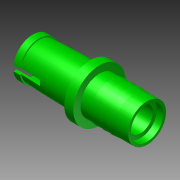
# Autodesk Inventor part: T9 Axle
Saved by Autodesk Inventor 2015 (Build 190159000, 159)
## iProperties
Created: 2012-02-20
Part Number: T9 Axle
Material: Generic
Document SubType Name: Modeling
Designer: Thom Tremblay
Density: 1 g/cm^3
Appearance: Dark Green
Author: Thom Tremblay
Autodesk Inventor part; units mm, degrees
ref_plane "YZ Plane" through (0, 0, 0) normal (1, 0, 0) x (0, 1, 0)
ref_plane "XZ Plane" through (0, 0, 0) normal (0, 1, 0) x (-1, 0, 0)
ref_plane "XY Plane" through (0, 0, 0) normal (0, 0, 1) x (1, 0, 0)
sketch "Sketch1" plane through (0, 0, 0) normal (0, 0, 1) x (1, 0, 0)
  line L0 (0, 0) -> (1.778, 0)
  line L1 (1.778, 0) -> (1.778, 5.08)
  line L2 (1.778, 5.08) -> (0, 5.08)
  line L3 (0, 5.08) -> (0, 0)
  line L4 (1.778, 0) -> (11.049, 0)
  line L5 (11.049, 0) -> (11.049, 3.683)
  line L6 (11.049, 3.683) -> (1.778, 3.683)
  line L7 (1.778, 3.683) -> (1.778, 0)
  line L8 (8.509, 3.683) -> (6.985, 3.81)
  line L9 (6.985, 3.81) -> (6.985, 3.683)
  line L10 (6.985, 3.683) -> (5.461, 3.81)
  line L11 (5.461, 3.81) -> (5.461, 3.683)
  line L12 (5.461, 3.683) -> (3.937, 3.81)
  line L13 (3.937, 3.81) -> (3.937, 3.683)
  line L14 (0, 0) -> (0, 3.1252)
  line L15 (0, 3.81) -> (0.889, 3.81) construction
  line L16 (0, 3.81) -> (0, 0)
  arc A0 (0, 3.81) -> (-9.906, 3.556) centre (0, -189.484) ccw
  line L17 (-9.906, 3.556) -> (-9.906, 3.81)
  line L18 (-9.906, 3.81) -> (-11.176, 3.81)
  line L19 (-11.176, 3.81) -> (-11.176, 0)
  line L20 (-11.176, 0) -> (0, 0)
  dimension "d0" = 1.778
  dimension "d1" = 10.16
  dimension "d2" = 9.271
  dimension "d3" = 7.366
  dimension "d4" = 7.62
  dimension "d5" = 2.54
  dimension "d6" = 1.524
  dimension "d7" = 7.62
  dimension "d8" = 7.62
  dimension "d9" = 11.176
  dimension "d10" = 7.112
  dimension "d11" = 1.27
  constraints: 42 end point, 8 parallel, 7 perpendicular, 6 point on line, 2 collinear, 2 horizontal, 2 horizontal alignment, 2 point on circle, 1 centre point, 1 tangent
  measures "d0" distance of L1.end L2.end
  measures "d1" diameter of L2 L0
  measures "d2" distance of L5.end L6.end
  measures "d3" diameter of L6 L4
  measures "d4" diameter of L8.end L4
  measures "d5" distance of L5.end L8.start
  measures "d6" horizontal distance of L8.start L8.end
  measures "d7" diameter of L18 L20
  measures "d8" diameter of L15 L20
  measures "d9" distance of L19.end L0.start
  measures "d10" diameter of L17.start L20
  measures "d11" distance of L17.end L18.end
revolve "Revolution1" add sketch "Sketch1" angle 360 about axis through (-11.176, 0, 0) along (1, 0, 0)
sketch "Sketch2" plane through (0, 0, 0) normal (0, 0, 1) x (1, 0, 0)
  line L0 (-11.176, 0.508) -> (-6.096, 0.508)
  line L1 (-6.096, 0.508) -> (-6.096, -0.508)
  line L2 (-6.096, -0.508) -> (-11.176, -0.508)
  line L3 (-11.176, -0.508) -> (-11.176, 0.508)
  line L4 (-11.176, -3.81) -> (-11.176, 3.81) construction
  point P0 (0, 0)
  point P1 (-11.176, 0)
  dimension "d13" = 1.016
  dimension "d14" = 5.08
  constraints: 8 end point, 2 midpoint, 2 parallel, 1 horizontal, 1 perpendicular
  measures "d13" distance of L2.end L0.start
  measures "d14" distance of L0.start L0.end
extrude "Extrusion1" cut sketch "Sketch2" along normal through all both and the other way through all
hole "Hole1" at (-11.176, 0, 0) direction (1, 0, 0) diameter 4.7625 depth 11.1125 counterbore diameter 6.35 counterbore depth 6.35
hole "Hole2" at (11.049, 0, 0) direction (-1, 0, 0) diameter 4.7625 depth 9.525 counterbore diameter 6.35 counterbore depth 1.27
equation "\"d8\" = d7"
body "Solid1"
